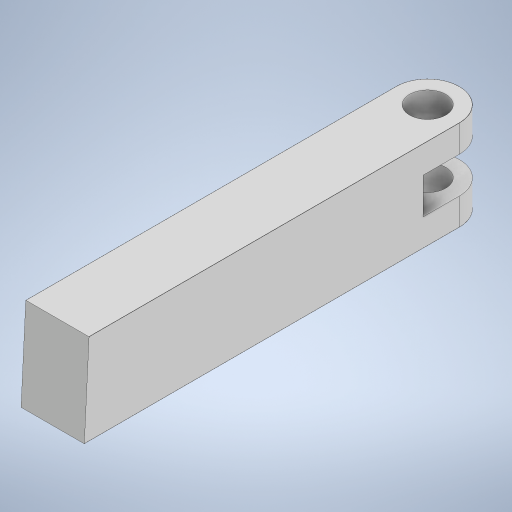
# Autodesk Inventor part: Schneidstempel
Saved by Autodesk Inventor 2023.2 (Build 272271030, 271C)
## iProperties
Created: 2023-02-11
Part Number: Schneidstempel
Material: Generic
Document SubType Name: Modeling
Designer: Ayush
Density: 1 g/cm^3
Appearance: Default
Author: Ayush
Autodesk Inventor part; units mm, degrees
ref_plane "YZ Plane" through (0, 0, 0) normal (1, 0, 0) x (0, 1, 0)
ref_plane "XZ Plane" through (0, 0, 0) normal (0, 1, 0) x (-1, 0, 0)
ref_plane "XY Plane" through (0, 0, 0) normal (0, 0, 1) x (1, 0, 0)
sketch "Sketch1" plane through (0, 0, 0) normal (0, 1, 0) x (-1, 0, 0)
  line L0 (-7, 0) -> (-7, -45)
  line L1 (-7, 0) -> (-7, 45)
  line L2 (-7, 45) -> (7, 45)
  line L3 (7, 45) -> (7, -45)
  circle A0 centre (0, -38) radius 4
  line L4 (7, -45) -> (-7, -45)
  point P0 (0, 0)
  dimension "d4" = 45
  dimension "d5" = 45
  dimension "d6" = 14
  dimension "d7" = 90
  dimension "d8" = 8
  dimension "d9" = 7
  constraints: 10 end point, 3 vertical, 1 centre point, 1 horizontal
  measures "d4" distance of L0.start L0.end
  measures "d5" distance of L0.start L1.end
  measures "d6" distance of L1.end L2.end
  measures "d7" distance of L2.end L3.end
  measures "d8" diameter of A0
  measures "d9" distance from line of A0.centre L4
extrude "Extrusion1" add sketch "Sketch1" along normal blind 6
fillet "Fillet1" radius 7 2 edges at (7, 3, -45) (-7, 3, -45)
sketch "Sketch2" plane through (0, 6, 0) normal (0, 1, 0) x (1, 0, 0)
  line L0 (-7, 38) -> (-7, -45) projected
  line L1 (-7, 30) -> (7, 30)
  line L2 (7, -45) -> (7, 38) projected
  arc A0 (7, 38) -> (-7, 38) centre (0, 38) ccw projected
  line L3 (-7, 30) -> (-7, -45)
  line L4 (-7, -45) -> (7, -45) projected
  line L5 (-7, -45) -> (7, -45)
  line L6 (7, -45) -> (7, 30)
  point P0 (0, 0)
  point P1 (0, 30)
  point P2 (0, 45)
  dimension "d13" = 15
  constraints: 8 end point, 2 point on line, 1 collinear, 1 horizontal, 1 midpoint, 1 perpendicular, 1 point on circle
  measures "d13" distance of point (0, 30) point (0, 45)
extrude "Extrusion2" add sketch "Sketch2" along normal blind 8 contours L1 L2 L4 L0
sketch "Sketch3" plane through (0, 14, 0) normal (0, 1, 0) x (1, 0, 0)
  line L0 (-7, -45) -> (7, -45) projected
  line L1 (-7, -45) -> (-7, 45)
  line L2 (-7, 38) -> (-7, -45) projected
  line L3 (-7, 45) -> (7, 45)
  line L4 (7, -45) -> (7, 38) projected
  line L5 (7, 45) -> (7, -45)
  line L6 (7, -45) -> (-7, -45)
  circle A0 centre (0, 38) radius 4
  point P0 (0, 0)
  dimension "d16" = 90
  dimension "d17" = 8
  dimension "d18" = 7
  constraints: 8 end point, 3 collinear, 1 centre point, 1 horizontal
  measures "d16" distance of L0.start L1.end
  measures "d17" diameter of A0
  measures "d18" distance from line of L3 A0.centre
extrude "Extrusion3" add sketch "Sketch3" along normal blind 6
fillet "Fillet2" radius 7 2 edges at (7, 17, -45) (-7, 17, -45)
draft "FaceDraft1" angle 3 pull direction (0, 1, 0) faces at (2.3333, 13.3333, 45) fixed edges at (0, 0, 45)
chamfer "Chamfer1" distance 0.02 angle 45 3 edges at (7, 20, 2.9759) (4.9498, 20, -42.9498) (-7, 20, 2.9759)
chamfer "Chamfer2" distance 0.02 angle 45 3 edges at (7, 0, 3.5) (4.9498, 0, -42.9498) (-7, 0, 3.4999)
chamfer "Chamfer3" distance 0.02 angle 45 3 edges at (6.98, 20, 2.9759) (4.9356, 20, -42.9356) (-6.98, 20, 2.9759)
chamfer "Chamfer4" distance 0.02 angle 45 3 edges at (-7, 0.02, 3.4994) (4.9498, 0.02, -42.9498) (7, 0.02, 3.4994)
body "Solid1"
